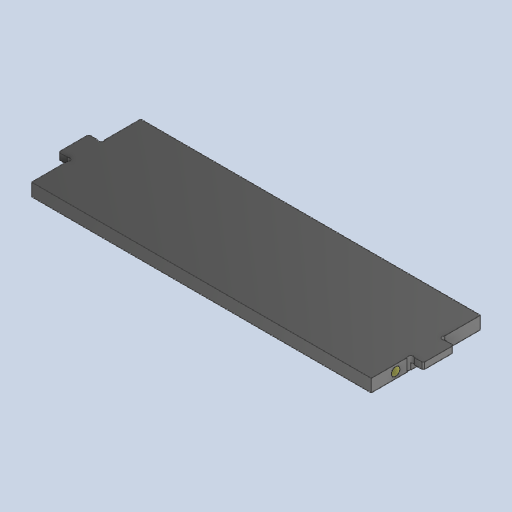
# Autodesk Inventor part: Cockpit_battery_bottom_frame
Saved by Autodesk Inventor 2022 (Build 260153000, 153)
## iProperties
Part Number: Cockpit_battery_bottom_frame
Material: アセタール樹脂、黒
Document SubType Name: Modeling
Designer: Masato Kubotera
Density: 1.425 g/cm^3
Appearance: 滑らか - 黒
Description: POM T5
Mass: 15.4882 g
Surface Area: 160.685 cm^2
Volume: 10.8689 cm^3
Author: Masato Kubotera
Autodesk Inventor part; units mm, degrees
ref_plane "YZ Plane" through (0, 0, 0) normal (1, 0, 0) x (0, 1, 0)
derived "Cockpit_side_frame.ipt"
sketch "スケッチ2" plane through (0, 0, 0) normal (0, 1, 0) x (-1, 0, 0)
  line L0 (-23.5, -22.5) -> (-28.5, -27.5)
  line L1 (-28.5, -27.5) -> (-28.5, -91)
  line L2 (-28.5, -91) -> (-23.5, -96)
  line L3 (-23.5, -96) -> (34.25, -96)
  line L4 (36.25, -98) -> (36.25, -131)
  line L5 (36.25, -131) -> (41.25, -136)
  line L6 (41.25, -136) -> (86.5, -136)
  line L7 (91.5, -131) -> (91.5, -20)
  line L8 (91.5, -20) -> (89, -17.5)
  line L9 (89, -17.5) -> (83.25, -17.5)
  line L10 (83.25, -17.5) -> (83.25, -21.0151)
  line L11 (81.7651, -22.5) -> (76.9849, -22.5)
  line L12 (75.5, -21.0151) -> (75.5, -17.5)
  line L13 (75.5, -17.5) -> (67.5, -17.5)
  line L14 (67.5, -17.5) -> (67.5, -21.0151)
  line L15 (66.0151, -22.5) -> (-23.5, -22.5)
  line L16 (-25.25, -25) -> (-20.25, -25) construction
  line L17 (-20.25, -25) -> (-20.25, -93.5) construction
  line L18 (-20.25, -93.5) -> (-25.25, -93.5) construction
  line L19 (-25.25, -93.5) -> (-25.25, -25) construction
  line L20 (-26, -25) -> (-25.25, -25) construction
  line L21 (-25.25, -93.5) -> (-26, -93.5) construction
  line L22 (-26, -93.5) -> (-26, -25) construction
  line L23 (-20.25, -93.5) -> (83.25, -93.5) construction
  line L24 (-20.25, -88.5) -> (83.25, -88.5) construction
  line L25 (83.25, -22.5) -> (83.25, -90.5) construction
  line L26 (83.25, -90.5) -> (88.25, -90.5) construction
  line L27 (88.25, -90.5) -> (88.25, -22.5) construction
  line L28 (83.25, -88.5) -> (83.25, -93.5) construction
  line L29 (83.25, -91) -> (88.25, -91) construction
  line L30 (88.25, -91) -> (88.25, -133.5) construction
  line L31 (83.25, -91) -> (83.25, -133.5) construction
  line L32 (83.25, -133.5) -> (88.25, -133.5) construction
  line L33 (38.75, -133.5) -> (38.75, -128.5) construction
  line L34 (38.75, -128.5) -> (38.75, -93.5) construction
  line L35 (43.75, -93.5) -> (43.75, -128.5) construction
  line L36 (38.75, -128.5) -> (43.75, -128.5) construction
  line L37 (41.25, -128.5) -> (41.25, -93.5) construction
  line L38 (38.75, -128.5) -> (82.1145, -128.5) construction
  line L39 (82.1145, -128.5) -> (82.1145, -133.5) construction
  line L40 (82.1145, -133.5) -> (38.75, -133.5) construction
  line L41 (38.75, -131) -> (82.1145, -131) construction
  line L42 (85.75, -91) -> (85.75, -133.5) construction
  circle A0 centre (85.75, -131) radius 2
  arc A1 (83.25, -128.5) -> (88.25, -128.5) centre (85.75, -131) ccw construction
  line L43 (83.25, -91) -> (-20.25, -91) construction
  line L44 (41.25, -111) -> (43.75, -111) construction
  line L45 (60.4322, -128.5) -> (60.4322, -131) construction
  line L46 (41.2, -115.5651) -> (41.2, -106.4349)
  line L47 (43.8, -107.05) -> (43.8, -114.95)
  line L48 (43.8, -117.05) -> (41.2, -104.95) construction
  line L49 (41.2, -117.05) -> (43.8, -104.95) construction
  line L50 (56.4822, -128.45) -> (64.3822, -128.45)
  line L51 (64.9973, -131.05) -> (55.8672, -131.05)
  line L52 (54.3822, -128.45) -> (66.4822, -131.05) construction
  line L53 (66.4822, -128.45) -> (54.3822, -131.05) construction
  line L54 (41.25, -105) -> (43.75, -105) construction
  line L55 (41.25, -117) -> (43.75, -117) construction
  arc A2 (42.6849, -104.95) -> (41.2, -106.4349) centre (41.9425, -105.6925) ccw
  arc A3 (43.8, -107.05) -> (43.8, -104.95) centre (43.8, -106) ccw
  arc A4 (41.2, -115.5651) -> (42.6849, -117.05) centre (41.9425, -116.3075) ccw
  arc A5 (43.8, -117.05) -> (43.8, -114.95) centre (43.8, -116) ccw
  line L56 (54.4322, -131) -> (54.4322, -128.5) construction
  line L57 (66.4322, -128.5) -> (66.4322, -131) construction
  arc A6 (54.3822, -129.5651) -> (55.8672, -131.05) centre (55.1247, -130.3075) ccw
  arc A7 (56.4822, -128.45) -> (54.3822, -128.45) centre (55.4322, -128.45) ccw
  arc A8 (64.9973, -131.05) -> (66.4822, -129.5651) centre (65.7398, -130.3075) ccw
  arc A9 (66.4822, -128.45) -> (64.3822, -128.45) centre (65.4322, -128.45) ccw
  line L58 (54.3822, -129.5651) -> (54.3822, -128.45)
  line L59 (66.4822, -128.45) -> (66.4822, -129.5651)
  line L60 (42.6849, -104.95) -> (43.8, -104.95)
  line L61 (43.8, -117.05) -> (42.6849, -117.05)
  circle A10 centre (48.4322, -131) radius 1.6
  line L62 (88.25, -22.5) -> (88.25, -17.5) construction
  line L63 (89, -17.5) -> (89, -90.5) construction
  line L64 (89, -90.5) -> (88.25, -90.5) construction
  line L65 (-13.5, -82.5) -> (-13.5, -61)
  arc A11 (-13.5, -82.5) -> (-11.5, -84.5) centre (-11.5, -82.5) ccw
  line L66 (45.5, -84.5) -> (-11.5, -84.5)
  arc A12 (45.5, -84.5) -> (47.5, -82.5) centre (45.5, -82.5) ccw
  line L67 (47.5, -61) -> (47.5, -82.5)
  arc A13 (47.5, -61) -> (45.5, -59) centre (45.5, -61) ccw
  line L68 (-11.5, -59) -> (45.5, -59)
  arc A14 (-11.5, -59) -> (-13.5, -61) centre (-11.5, -61) ccw
  line L69 (31.5, -88.5) -> (31.5, -91) construction
  line L70 (85.75, -22.5) -> (85.75, -90.5) construction
  circle A15 centre (85.75, -34) radius 1.6
  circle A16 centre (85.75, -34) radius 3
  circle A17 centre (85.75, -79) radius 3
  circle A18 centre (85.75, -79) radius 1.6
  line L71 (88.25, -22.5) -> (83.25, -22.5) construction
  arc A19 (88.25, -91) -> (83.25, -91) centre (85.75, -131) ccw construction
  circle A20 centre (48.4322, -131) radius 3
  circle A21 centre (41.25, -99) radius 1.6
  circle A22 centre (41.25, -99) radius 3
  line L72 (6.5, -88.5) -> (6.5, -91) construction
  line L73 (56.5, -88.5) -> (56.5, -91) construction
  line L74 (55.0651, -91.05) -> (7.9349, -91.05)
  line L75 (6.45, -89.5651) -> (6.45, -88.45)
  line L76 (8.55, -88.45) -> (54.45, -88.45)
  line L77 (56.55, -88.45) -> (56.55, -89.5651)
  line L78 (56.55, -91.05) -> (6.45, -88.45) construction
  line L79 (6.45, -91.05) -> (56.55, -88.45) construction
  arc A23 (8.55, -88.45) -> (6.45, -88.45) centre (7.5, -88.45) ccw
  arc A24 (6.45, -89.5651) -> (7.9349, -91.05) centre (7.1925, -90.3075) ccw
  arc A25 (55.0651, -91.05) -> (56.55, -89.5651) centre (55.8075, -90.3075) ccw
  arc A26 (56.55, -88.45) -> (54.45, -88.45) centre (55.5, -88.45) ccw
  line L80 (-20.25, -41) -> (83.25, -41) construction
  line L81 (83.25, -36) -> (-20.25, -36) construction
  line L82 (-20.25, -36) -> (-20.25, -41) construction
  line L83 (-20.25, -38.5) -> (83.25, -38.5) construction
  line L84 (31.5, -41) -> (31.5, -36) construction
  line L85 (55.0651, -35.95) -> (7.9349, -35.95)
  line L86 (7.9349, -41.05) -> (55.0651, -41.05)
  line L87 (56.55, -35.95) -> (6.45, -41.05) construction
  line L88 (6.45, -35.95) -> (55.5877, -40.952) construction
  arc A27 (7.9349, -35.95) -> (6.45, -37.4349) centre (7.1925, -36.6925) ccw
  arc A28 (6.45, -39.5651) -> (7.9349, -41.05) centre (7.1925, -40.3075) ccw
  arc A29 (56.55, -37.4349) -> (55.0651, -35.95) centre (55.8075, -36.6925) ccw
  arc A30 (55.0651, -41.05) -> (56.55, -39.5651) centre (55.8075, -40.3075) ccw
  line L89 (6.5, -41) -> (6.5, -36) construction
  line L90 (56.5, -36) -> (56.5, -41) construction
  line L91 (6.45, -37.4349) -> (6.45, -39.5651)
  line L92 (56.55, -39.5651) -> (56.55, -37.4349)
  circle A31 centre (-1, -38.5) radius 1.6
  circle A32 centre (-1, -38.5) radius 3
  circle A33 centre (64, -38.5) radius 1.6
  circle A34 centre (64, -38.5) radius 3
  line L93 (-25.25, -49.25) -> (-26, -49.25) construction
  line L94 (-25.25, -69.25) -> (-26, -69.25) construction
  line L95 (-26, -59.25) -> (-25.25, -59.25) construction
  line L96 (-22.75, -25) -> (-22.75, -93.5) construction
  arc A35 (66.0151, -22.5) -> (67.5, -21.0151) centre (66.7575, -21.7575) ccw
  arc A36 (75.5, -21.0151) -> (76.9849, -22.5) centre (76.2425, -21.7575) ccw
  line L97 (59.75, -22.5) -> (59.75, -32.5) construction
  line L98 (59.75, -32.5) -> (83.25, -32.5) construction
  line L99 (83.25, -32.5) -> (83.25, -22.5) construction
  line L100 (71.5, -17.5) -> (71.5, -32.5) construction
  line L101 (63.5, -22.5) -> (63.5, -17.5) construction
  line L102 (79.5, -22.5) -> (79.5, -17.5) construction
  circle A37 centre (-22.75, -31.75) radius 1.6
  circle A38 centre (-22.75, -31.75) radius 3
  circle A39 centre (-22.75, -86.75) radius 1.6
  circle A40 centre (-22.75, -86.75) radius 3
  line L103 (67.5, -22.5) -> (75.5, -22.5)
  line L104 (88.25, -17.5) -> (52.5, -17.5) construction
  line L105 (52.5, -17.5) -> (52.5, -22.5) construction
  circle A41 centre (85.75, -98.5) radius 1.475
  circle A42 centre (85.75, -103.5) radius 1.475
  circle A43 centre (85.75, -108.5) radius 1.475
  line L106 (48.25, -93.5) -> (78.75, -93.5)
  line L107 (80.75, -95.5) -> (80.75, -124)
  line L108 (78.75, -126) -> (48.25, -126)
  line L109 (46.25, -124) -> (46.25, -95.5)
  arc A44 (48.25, -93.5) -> (46.25, -95.5) centre (48.25, -95.5) ccw
  arc A45 (46.25, -124) -> (48.25, -126) centre (48.25, -124) ccw
  arc A46 (78.75, -126) -> (80.75, -124) centre (78.75, -124) ccw
  arc A47 (80.75, -95.5) -> (78.75, -93.5) centre (78.75, -95.5) ccw
  arc A48 (36.25, -98) -> (34.25, -96) centre (34.25, -98) ccw
  circle A49 centre (-13.5, -55) radius 1.75
  circle A50 centre (-13.5, -55) radius 2
  line L110 (77.85, -78.65) -> (68.65, -78.65) construction
  line L111 (68.65, -78.65) -> (68.65, -64.85) construction
  line L112 (68.65, -64.85) -> (77.85, -64.85) construction
  line L113 (77.85, -64.85) -> (77.85, -78.65) construction
  line L114 (77.85, -78.65) -> (68.65, -64.85) construction
  line L115 (68.65, -78.65) -> (77.85, -64.85) construction
  line L116 (67.95, -64.2) -> (78.55, -64.2) construction
  line L117 (78.55, -64.2) -> (78.55, -79.3) construction
  line L118 (78.55, -79.3) -> (67.95, -79.3) construction
  line L119 (67.95, -79.3) -> (67.95, -64.2) construction
  line L120 (67.95, -64.2) -> (78.55, -79.3) construction
  line L121 (78.55, -64.2) -> (67.95, -79.3) construction
  line L122 (69.3849, -64.15) -> (77.1151, -64.15)
  line L123 (78.6, -65.6349) -> (78.6, -77.8651)
  line L124 (78.6, -79.35) -> (67.9, -64.15) construction
  line L125 (67.9, -79.35) -> (78.6, -64.15) construction
  line L126 (77.9, -78.7) -> (68.6, -64.8) construction
  line L127 (68.6, -78.7) -> (77.9, -64.8) construction
  arc A51 (69.3849, -64.15) -> (67.9, -65.6349) centre (68.6425, -64.8925) ccw
  arc A52 (70.0849, -64.8) -> (68.6, -66.2849) centre (69.3425, -65.5425) ccw
  line L128 (67.9, -71.75) -> (78.6, -71.75) construction
  line L129 (73.25, -64.15) -> (73.25, -78.7063) construction
  arc A53 (78.6, -65.6349) -> (77.1151, -64.15) centre (77.8575, -64.8925) ccw
  arc A54 (77.9, -66.2849) -> (76.4151, -64.8) centre (77.1575, -65.5425) ccw
  arc A55 (68.6, -77.2151) -> (70.0849, -78.7) centre (69.3425, -77.9575) ccw
  arc A56 (67.9, -77.8651) -> (69.3849, -79.35) centre (68.6425, -78.6075) ccw
  arc A57 (76.4151, -78.7) -> (77.9, -77.2151) centre (77.1575, -77.9575) ccw
  arc A58 (77.1151, -79.35) -> (78.6, -77.8651) centre (77.8575, -78.6075) ccw
  line L130 (70.0849, -64.8) -> (76.4151, -64.8)
  line L131 (77.9, -66.2849) -> (77.9, -77.2151)
  line L132 (67.9, -77.8651) -> (67.9, -65.6349)
  line L133 (68.6, -77.2151) -> (68.6, -66.2849)
  line L134 (76.4151, -78.7) -> (70.0849, -78.7)
  line L135 (77.1151, -79.35) -> (69.3849, -79.35)
  line L136 (-13.5, -71.75) -> (47.5, -71.75) construction
  line L137 (85.75, -56.5) -> (88.25, -56.5) construction
  line L138 (89, -54) -> (88.25, -54) construction
  line L139 (85.7, -69.45) -> (85.7, -43.55)
  line L140 (88.2835, -71.3588) -> (85.7, -41.45) construction
  line L141 (85.7, -71.55) -> (88.3, -41.45) construction
  arc A59 (85.7, -41.45) -> (85.7, -43.55) centre (85.7, -42.5) ccw
  arc A60 (88.3, -42.9349) -> (86.8151, -41.45) centre (87.5575, -42.1925) ccw
  arc A61 (85.7, -69.45) -> (85.7, -71.55) centre (85.7, -70.5) ccw
  arc A62 (86.8151, -71.55) -> (88.3, -70.0651) centre (87.5575, -70.8075) ccw
  line L142 (85.75, -41.5) -> (88.25, -41.5) construction
  line L143 (85.75, -71.5) -> (88.25, -71.5) construction
  arc A63 (89.25, -47.1801) -> (88.3, -46.1348) centre (88.2, -47.1801) ccw
  line L144 (89.25, -47.1801) -> (89.25, -65.8199)
  line L145 (88.25, -46.5) -> (89, -46.5) construction
  line L146 (88.25, -66.5) -> (89, -66.5) construction
  arc A64 (88.3, -66.8652) -> (89.25, -65.8199) centre (88.2, -65.8199) ccw
  line L147 (88.3, -42.9349) -> (88.3, -46.1348)
  line L148 (88.3, -66.8652) -> (88.3, -70.0651)
  line L149 (86.8151, -71.55) -> (85.7, -71.55)
  line L150 (85.7, -41.45) -> (86.8151, -41.45)
  line L151 (86.5, -136) -> (91.5, -131)
  arc A65 (81.7651, -22.5) -> (83.25, -21.0151) centre (82.5075, -21.7575) ccw
  circle A66 centre (85.75, -93.5) radius 2
  circle A67 centre (85.75, -93.5) radius 4 construction
  arc A68 (-24.15, -49.25) -> (-26.25, -49.25) centre (-25.2, -49.25) ccw
  line L152 (-26, -49.25) -> (-26.25, -49.25) construction
  line L153 (-26.25, -49.25) -> (-26.25, -69.25)
  line L154 (-24.15, -49.25) -> (-24.15, -69.25)
  arc A69 (-26.25, -69.25) -> (-24.15, -69.25) centre (-25.2, -69.25) ccw
  point P0 (0, 0)
  point P1 (-25.7227, -96)
  point P2 (-23.5, -22.5)
  point P3 (42.5, -111)
  point P4 (60.4322, -129.75)
  point P5 (31.5, -89.75)
  point P6 (31.5, -38.5)
  point P7 (6.45, -41.05)
  point P8 (52.5, -22)
  point P9 (73.25, -71.75)
  point P10 (73.25, -71.75)
  point P11 (87, -56.5)
  dimension "d1" = 128.5
  dimension "d2" = 5
  dimension "d3" = 2.5
  measures "d1" vertical distance of L33.end point (0, 0)
  measures "d2" distance of L33.start L33.end
  measures "d3" distance of L56.start L56.end
ref_plane "作業平面1" through (0, 0, -128.5) normal (0, 0, 1) x (1, 0, 0)
sketch "スケッチ3" plane through (0, 0, -128.5) normal (0, 0, 1) x (1, 0, 0)
  line L0 (-38.75, -135) -> (-38.75, 0)
  line L1 (-82.1145, 0) -> (-82.1145, -135)
  line L2 (-66.4322, 1.4849) -> (-66.4322, 5)
  line L3 (-66.4322, 5) -> (-54.4322, 5)
  line L4 (-60.4322, -135) -> (-60.4322, 0) construction
  line L5 (-82.1145, -67.5) -> (-38.75, -67.5) construction
  arc A0 (-67.9172, 0) -> (-66.4322, 1.4849) centre (-67.1747, 0.7425) ccw
  line L6 (-67.9172, 0) -> (-82.1145, 0)
  line L7 (-54.4322, 1.4849) -> (-54.4322, 5)
  arc A1 (-54.4322, 1.4849) -> (-52.9473, 0) centre (-53.6898, 0.7425) ccw
  line L8 (-52.9473, 0) -> (-38.75, 0)
  line L9 (-38.75, 0) -> (-52.9473, 0)
  line L10 (-54.4322, 0) -> (-66.4322, 0)
  line L11 (-66.4322, -136.4849) -> (-66.4322, -140)
  line L12 (-66.4322, -140) -> (-54.4322, -140)
  arc A2 (-66.4322, -136.4849) -> (-67.9172, -135) centre (-67.1747, -135.7425) ccw
  line L13 (-67.9172, -135) -> (-82.1145, -135)
  line L14 (-52.9473, -135) -> (-38.75, -135)
  arc A3 (-52.9473, -135) -> (-54.4322, -136.4849) centre (-53.6898, -135.7425) ccw
  line L15 (-54.4322, -136.4849) -> (-54.4322, -140)
  line L16 (-54.4322, -135) -> (-66.4322, -135)
  line L17 (-53.6145, -14) -> (-43.25, -14)
  line L18 (-41.25, -12) -> (-41.25, -6)
  line L19 (-43.25, -4) -> (-53.6145, -4)
  line L20 (-55.6145, -6) -> (-55.6145, -12)
  line L21 (-41.25, -116.5) -> (-41.25, -18.5)
  line L22 (-43.25, -16.5) -> (-53.7545, -16.5)
  line L23 (-55.7525, -18.4112) -> (-57.9303, -67.4112)
  line L24 (-58.4342, -22.4442) -> (-58.1164, -15.2944)
  line L25 (-58.1145, -15.2056) -> (-58.1145, -6)
  line L26 (-60.1145, -4) -> (-60.75, -4)
  line L27 (-67.25, -14) -> (-77.6145, -14)
  line L28 (-79.6145, -12) -> (-79.6145, -6)
  line L29 (-77.6145, -4) -> (-67.25, -4)
  line L30 (-65.25, -6) -> (-65.25, -12)
  line L31 (-79.6145, -116.5) -> (-79.6145, -18.5)
  line L32 (-77.6145, -16.5) -> (-67.11, -16.5)
  line L33 (-65.112, -18.4112) -> (-62.9342, -67.4112)
  line L34 (-62.4303, -22.4442) -> (-62.748, -15.2944)
  line L35 (-62.75, -15.2056) -> (-62.75, -6)
  line L36 (-43.25, -118.5) -> (-53.7545, -118.5)
  line L37 (-55.7525, -116.5888) -> (-57.9303, -67.5888)
  line L38 (-65.112, -116.5888) -> (-62.9342, -67.5888)
  line L39 (-77.6145, -118.5) -> (-67.11, -118.5)
  line L40 (-48.4322, -4) -> (-48.4322, 0) construction
  arc A4 (-43.25, -118.5) -> (-41.25, -116.5) centre (-43.25, -116.5) ccw
  arc A5 (-55.7525, -116.5888) -> (-53.7545, -118.5) centre (-53.7545, -116.5) ccw
  arc A6 (-67.11, -118.5) -> (-65.112, -116.5888) centre (-67.11, -116.5) ccw
  arc A7 (-79.6145, -116.5) -> (-77.6145, -118.5) centre (-77.6145, -116.5) ccw
  arc A8 (-62.9342, -67.5888) -> (-62.9342, -67.4112) centre (-64.9322, -67.5) ccw
  arc A9 (-57.9303, -67.4112) -> (-57.9303, -67.5888) centre (-55.9322, -67.5) ccw
  arc A10 (-62.4303, -22.4442) -> (-58.4342, -22.4442) centre (-60.4322, -22.3554) ccw
  arc A11 (-65.112, -18.4112) -> (-67.11, -16.5) centre (-67.11, -18.5) ccw
  arc A12 (-77.6145, -16.5) -> (-79.6145, -18.5) centre (-77.6145, -18.5) ccw
  arc A13 (-53.7545, -16.5) -> (-55.7525, -18.4112) centre (-53.7545, -18.5) ccw
  arc A14 (-41.25, -18.5) -> (-43.25, -16.5) centre (-43.25, -18.5) ccw
  arc A15 (-43.25, -14) -> (-41.25, -12) centre (-43.25, -12) ccw
  arc A16 (-41.25, -6) -> (-43.25, -4) centre (-43.25, -6) ccw
  arc A17 (-53.6145, -4) -> (-55.6145, -6) centre (-53.6145, -6) ccw
  arc A18 (-55.6145, -12) -> (-53.6145, -14) centre (-53.6145, -12) ccw
  arc A19 (-58.1164, -15.2944) -> (-58.1145, -15.2056) centre (-60.1145, -15.2056) ccw
  arc A20 (-58.1145, -6) -> (-60.1145, -4) centre (-60.1145, -6) ccw
  arc A21 (-60.75, -4) -> (-62.75, -6) centre (-60.75, -6) ccw
  arc A22 (-62.75, -15.2056) -> (-62.748, -15.2944) centre (-60.75, -15.2056) ccw
  arc A23 (-67.25, -14) -> (-65.25, -12) centre (-67.25, -12) ccw
  arc A24 (-65.25, -6) -> (-67.25, -4) centre (-67.25, -6) ccw
  arc A25 (-79.6145, -12) -> (-77.6145, -14) centre (-77.6145, -12) ccw
  arc A26 (-77.6145, -4) -> (-79.6145, -6) centre (-77.6145, -6) ccw
  line L41 (-53.6145, -121) -> (-43.25, -121)
  line L42 (-43.25, -131) -> (-53.6145, -131)
  line L43 (-55.6145, -129) -> (-55.6145, -123)
  line L44 (-58.4342, -112.5558) -> (-58.1164, -119.7056)
  line L45 (-58.1145, -119.7944) -> (-58.1145, -129)
  line L46 (-62.4303, -112.5558) -> (-62.748, -119.7056)
  line L47 (-62.75, -119.7944) -> (-62.75, -129)
  line L48 (-67.25, -121) -> (-77.6145, -121)
  line L49 (-65.25, -129) -> (-65.25, -123)
  line L50 (-79.6145, -123) -> (-79.6145, -129)
  line L51 (-77.6145, -131) -> (-67.25, -131)
  arc A27 (-58.4342, -112.5558) -> (-62.4303, -112.5558) centre (-60.4322, -112.6446) ccw
  arc A28 (-41.25, -123) -> (-43.25, -121) centre (-43.25, -123) ccw
  arc A29 (-43.25, -131) -> (-41.25, -129) centre (-43.25, -129) ccw
  arc A30 (-55.6145, -129) -> (-53.6145, -131) centre (-53.6145, -129) ccw
  arc A31 (-53.6145, -121) -> (-55.6145, -123) centre (-53.6145, -123) ccw
  arc A32 (-58.1145, -119.7944) -> (-58.1164, -119.7056) centre (-60.1145, -119.7944) ccw
  arc A33 (-60.1145, -131) -> (-58.1145, -129) centre (-60.1145, -129) ccw
  arc A34 (-62.75, -129) -> (-60.75, -131) centre (-60.75, -129) ccw
  arc A35 (-62.748, -119.7056) -> (-62.75, -119.7944) centre (-60.75, -119.7944) ccw
  arc A36 (-65.25, -123) -> (-67.25, -121) centre (-67.25, -123) ccw
  arc A37 (-67.25, -131) -> (-65.25, -129) centre (-67.25, -129) ccw
  arc A38 (-77.6145, -121) -> (-79.6145, -123) centre (-77.6145, -123) ccw
  arc A39 (-79.6145, -129) -> (-77.6145, -131) centre (-77.6145, -129) ccw
  line L52 (-41.25, -123) -> (-41.25, -129)
  line L53 (-60.1145, -131) -> (-60.75, -131)
  point P0 (0, 0)
  point P1 (-60.4322, -67.5)
  point P2 (-54.4322, -135)
  point P3 (-55.6145, -14)
  point P4 (-41.25, -4)
  point P5 (-41.25, -14)
  point P6 (-55.6145, -4)
  point P7 (-41.25, -118.5)
  point P8 (-41.25, -16.5)
  point P9 (-55.6676, -16.5)
  point P10 (-57.9342, -67.5)
  point P11 (-60.4322, -67.4)
  point P12 (-58.1145, -15.25)
  point P13 (-58.1145, -4)
  point P14 (-65.25, -14)
  point P15 (-79.6145, -4)
  point P16 (-79.6145, -14)
  point P17 (-65.25, -4)
  point P18 (-79.6145, -16.5)
  point P19 (-65.1969, -16.5)
  point P20 (-62.9303, -67.5)
  point P21 (-62.75, -15.25)
  point P22 (-62.75, -4)
  point P23 (-41.25, -118.5)
  point P24 (-55.6676, -118.5)
  point P25 (-65.1969, -118.5)
  point P26 (-79.6145, -118.5)
  dimension "d5" = 135
  dimension "d7" = 1.05
  dimension "d8" = 5
  dimension "d20" = 4
  dimension "d21" = 2.5
  dimension "d22" = 2.5
  dimension "d23" = 10
  dimension "d24" = 11.25
  dimension "d25" = 2.5
  dimension "d26" = 2.5
  dimension "d27" = 2
  dimension "d28" = 5
  constraints: 108 end point, 83 point on circle, 67 symmetric about line, 54 point on line, 46 tangent, 40 centre point, 22 equal radius, 7 perpendicular, 6 midpoint, 4 parallel, 3 collinear, 2 coincident, 2 vertical, 1 horizontal, 16 other
  measures "d5" distance of L1.start L1.end
  measures "d7" radius of A0
  measures "d8" distance between parallel lines of L3 L10
  measures "d20" distance between parallel lines of L8 L19
  measures "d21" distance between parallel lines of L0 L18
  measures "d22" distance between parallel lines of L22 L17
  measures "d23" distance of point (-41.25, -14) point (-41.25, -4)
  measures "d24" distance of point (-58.114, -15.25) point (-58.114, -4)
  measures "d25" distance between parallel lines of L23 L24
  measures "d26" distance between parallel lines of L20 L25
  measures "d27" radius of A4
extrude "押し出し1" add sketch "スケッチ3" against normal blind 5 contours L14 A3 L16 A2 L13 L1 L6 A0 L10 A1 L8 L0
extrude "押し出し2" add sketch "スケッチ3" against normal blind 2.5 contours A3 L15 L12 L11 A2 L16 | L10 A0 L2 L3 L7 A1
hole "穴1" at (-48.4322, 0, -131) direction (0, -1, 0) diameter 3.4587 depth 4 thread size "M4x0.5" class "6H" standard "ANSI Metric M Profile"
ref_plane "作業平面2" through (-38.75, -67.5, -128.5) normal (0, 1, 0) x (1, 0, 0)
mirror "ミラー1" about plane through (-38.75, -67.5, -128.5) normal (0, 1, 0) of "穴1"
extrude "押し出し3" add sketch "スケッチ3" against normal blind 0.5 contours A18 L20 A17 L19 A16 L18 A15 L17 | A4 L36 A5 L37 A9 L23 A13 L22 A14 L21 | A10 L34 A22 L35 A21 L26 A20 L25 A19 L24 | L27 A25 L28 A26 L29 A24 L30 A23 | L31 A12 L32 A11 L33 A8 L38 A6 L39 A7 | L41 A28 L52 A29 L42 A30 L43 A31 | L44 A32 L45 A33 L53 A34 L47 A35 L46 A27 | A36 L49 A37 L51 A39 L50 A38 L48
chamfer "面取り1" distance 0.5 angle 45 4 edges at (-66.4322, -140, -129.75) (-54.4322, -140, -129.75) (-66.4322, 5, -129.75) (-54.4322, 5, -129.75)
equation "\"d22\" = d21"
equation "\"d24\" = d23 + 0.5 * d22"
equation "\"d25\" = d21"
equation "\"d26\" = d21"
equation "\"d28\" = 2 * d21"
equation "\"d9\" = d2"
equation "\"d11\" = d3"
equation "\"d4\" = -d1"
